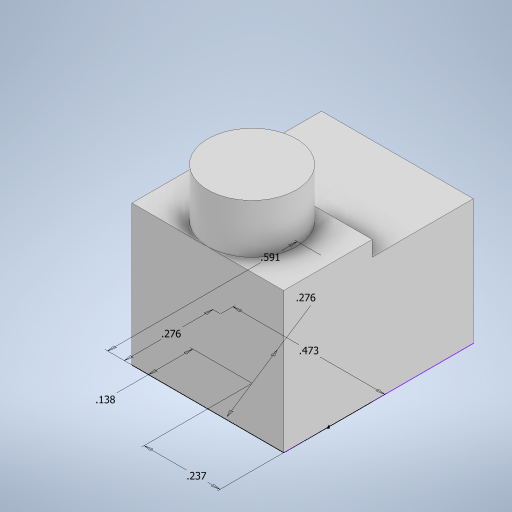
# Autodesk Inventor part: Audio_jack
Saved by Autodesk Inventor 2023 (Build 270158000, 158)
## iProperties
Created: 2022-12-07
Part Number: Audio_jack
Material: Generic
Document SubType Name: Modeling
Designer: spfow
Density: 1 g/cm^3
Appearance: Default
Author: spfow
Autodesk Inventor part; units mm, degrees
ref_plane "YZ Plane" through (0, 0, 0) normal (1, 0, 0) x (0, 1, 0)
ref_plane "XZ Plane" through (0, 0, 0) normal (0, 1, 0) x (-1, 0, 0)
ref_plane "XY Plane" through (0, 0, 0) normal (0, 0, 1) x (1, 0, 0)
sketch "Sketch1" plane through (0, 0, 0) normal (0, 1, 0) x (-1, 0, 0)
  line L0 (0, 0) -> (12.0142, 0)
  line L1 (12.0142, 0) -> (12.0142, -7.0104)
  line L2 (12.0142, -7.0104) -> (0, -7.0104)
  line L3 (0, -7.0104) -> (0, 0)
  circle A0 centre (6.0071, -3.5052) radius 3.5052
  line L4 (12.0142, 0) -> (0, 0)
  line L5 (0, 0) -> (0, -15.0114)
  line L6 (0, -15.0114) -> (12.0142, -15.0114)
  line L7 (12.0142, -15.0114) -> (12.0142, 0)
  point P0 (0, -3.5052)
  point P1 (6.0071, -7.0104)
  point P2 (6.0071, 0)
  dimension "d0" = 12.0142
  dimension "d1" = 7.0104
  dimension "d2" = 3.5052
  dimension "d3" = 6.0071
  dimension "d4" = 7.0104
  dimension "d5" = 15.0114
  constraints: 16 end point, 4 parallel, 2 horizontal, 2 perpendicular, 1 centre point, 1 midpoint
  measures "d0" distance of L1.end L2.end
  measures "d1" distance of L0.end L1.end
  measures "d2" distance from line of L0 A0.centre
  measures "d3" distance of point (0, -3.505) A0.centre
  measures "d4" diameter of A0
  measures "d5" distance of L6.end L0.end
extrude "Extrusion1" add sketch "Sketch1" along normal blind 9.906 contours L2 L7 L6 L5
extrude "Extrusion2" add sketch "Sketch1" along normal blind 11.1125 contours L0 A0 L2 L3 | L0 L1 L2 A0
extrude "Extrusion3" add sketch "Sketch1" along normal blind 15.0114 contours A0
body "Solid1"
